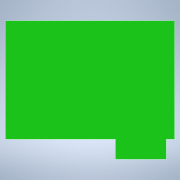
# Autodesk Inventor part: Pared_caja_reduccion_frontal
Saved by Autodesk Inventor 2022 (Build 260153000, 153)
## iProperties
Created: 2022-02-27
Part Number: Pared_caja_reduccion_frontal
Material: Generic
Document SubType Name: Modeling
Designer: Home
Density: 1 g/cm^3
Appearance: Dark Green
Author: Home
Autodesk Inventor part; units mm, degrees
ref_plane "YZ Plane" through (0, 0, 0) normal (1, 0, 0) x (0, 1, 0)
ref_plane "XZ Plane" through (0, 0, 0) normal (0, 1, 0) x (-1, 0, 0)
ref_plane "XY Plane" through (0, 0, 0) normal (0, 0, 1) x (1, 0, 0)
sketch "Sketch2" plane through (0, 0, 0) normal (0, 1, 0) x (-1, 0, 0)
  line L0 (25, -17.5) -> (-25, -17.5)
  line L1 (-25, -17.5) -> (-25, 17.5)
  line L2 (25, -17.5) -> (-25, 17.5) construction
  line L3 (-25, -17.5) -> (25, 17.5) construction
  line L4 (-22.5, 17.5) -> (-7.5, 17.5)
  line L5 (-7.5, 17.5) -> (-7.5, 23.5)
  line L6 (-7.5, 23.5) -> (-22.5, 23.5)
  line L7 (-22.5, 23.5) -> (-22.5, 17.5)
  line L8 (25, -17.5) -> (25, 17.5)
  line L9 (25, 17.5) -> (-25, 17.5)
  point P0 (0, 0)
  point P1 (0, 0)
  point P2 (-7.5, 17.5)
  dimension "d0" = 50
  dimension "d1" = 35
  dimension "d58" = 2.5
  dimension "d59" = 15
  dimension "d60" = 6
  constraints: 20 end point, 4 perpendicular, 3 midpoint, 2 horizontal, 2 parallel, 1 collinear
  measures "d0" distance of L1.end L3.end
  measures "d1" distance of L0.end L1.end
  measures "d58" distance between parallel lines of L1 L7
  measures "d59" distance of L5.end L6.end
  measures "d60" distance of L4.end L5.end
extrude "Extrusion12" add sketch "Sketch2" along normal blind 6
sketch "Sketch7" plane through (0, 6, 0) normal (0, 1, 0) x (1, 0, 0)
  line L0 (25, -17.5) -> (25, 17.5) projected
  line L1 (-25, -17.5) -> (7.5, -17.5) projected
  point P0 (0, 0)
extrude "Extrusion13" [suppressed]
body "Solid5"
